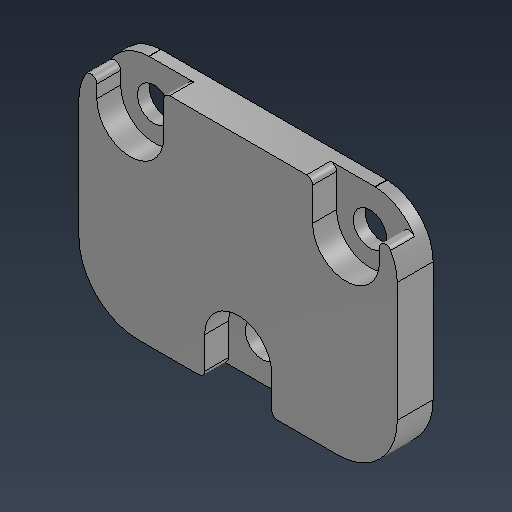
# Autodesk Inventor part: LunasCover
Saved by Autodesk Inventor 2026.2 (Build 302298010, 298A)
## iProperties
Created: 2026-04-20
Part Number: LunasCover
Material: Nylon 6/6
Document SubType Name: Modeling
Designer: szymo
Density: 1.13 g/cm^3
Appearance: Nylon 6(1)
Author: szymo
Autodesk Inventor part; units mm, degrees
ref_plane "YZ Plane" through (0, 0, 0) normal (1, 0, 0) x (0, 1, 0)
ref_plane "XZ Plane" through (0, 0, 0) normal (0, 1, 0) x (-1, 0, 0)
ref_plane "XY Plane" through (0, 0, 0) normal (0, 0, 1) x (1, 0, 0)
sketch "Sketch1" plane through (0, 0, 0) normal (0, 0, 1) x (1, 0, 0)
  circle A0 centre (0.0056, -6.3497) radius 1 projected
  circle A1 centre (-9.0264, 6.2307) radius 1 projected
  circle A2 centre (9.0376, 6.2307) radius 1 projected
  line L0 (9.4418, 9.5) -> (-9.4418, 9.5) projected
  arc A3 (-9.4806, 9.497) -> (-9.4418, 9.5) centre (-9.5, 9.9966) ccw projected
  arc A4 (-9.4806, 9.497) -> (-13.325, 5.5) centre (-9.325, 5.5) ccw projected
  line L1 (-13.325, -4.5) -> (-13.325, 5.5) projected
  arc A5 (-13.325, -4.5) -> (-8.325, -9.5) centre (-8.325, -4.5) ccw projected
  line L2 (8.325, -9.5) -> (-8.325, -9.5) projected
  arc A6 (8.325, -9.5) -> (13.325, -4.5) centre (8.325, -4.5) ccw projected
  line L3 (13.325, 5.5) -> (13.325, -4.5) projected
  arc A7 (13.325, 5.5) -> (9.4806, 9.497) centre (9.325, 5.5) ccw projected
  arc A8 (9.4418, 9.5) -> (9.4806, 9.497) centre (9.5, 9.9966) ccw projected
  point P0 (0, 0)
extrude "Extrusion1" add sketch "Sketch1" along normal blind 3
sketch "Sketch2" plane through (0, 0, 3) normal (0, 0, -1) x (-1, 0, 0)
  circle A0 centre (9.0264, 6.2307) radius 1 projected
  circle A1 centre (-0.0056, -6.3497) radius 1 projected
  circle A2 centre (-9.0376, 6.2307) radius 1 projected
  point P0 (0, 0)
hole "Hole1" at (-9.0264, 6.2307, 3) at (0.0056, -6.3497, 3) at (9.0376, 6.2307, 3) direction (0, 0, -1) diameter 2.8 depth 12 counterbore diameter 5.6 counterbore depth 2
sketch "Sketch3" plane through (0, 0, 3) normal (0, 0, 1) x (1, 0, 0)
  circle A0 centre (9.0376, 6.2307) radius 2.8 projected
  circle A1 centre (0.0056, -6.3497) radius 2.8 projected
  circle A2 centre (-9.0264, 6.2307) radius 2.8 projected
  arc A3 (9.4418, 9.5) -> (9.4806, 9.497) centre (9.5, 9.9966) ccw projected
  line L0 (9.4418, 9.5) -> (-9.4418, 9.5) projected
  arc A4 (-9.4806, 9.497) -> (-9.4418, 9.5) centre (-9.5, 9.9966) ccw projected
  arc A5 (-9.4806, 9.497) -> (-13.325, 5.5) centre (-9.325, 5.5) ccw projected
  line L1 (-13.325, 5.5) -> (-13.325, -4.5) projected
  arc A6 (-13.325, -4.5) -> (-8.325, -9.5) centre (-8.325, -4.5) ccw projected
  line L2 (-8.325, -9.5) -> (8.325, -9.5) projected
  arc A7 (8.325, -9.5) -> (13.325, -4.5) centre (8.325, -4.5) ccw projected
  line L3 (13.325, -4.5) -> (13.325, 5.5) projected
  arc A8 (13.325, 5.5) -> (9.4806, 9.497) centre (9.325, 5.5) ccw projected
  line L4 (-6.2264, 6.2307) -> (-6.2264, 9.5)
  line L5 (-11.8264, 6.2307) -> (-11.8264, 8.6214)
  circle A9 centre (-9.0264, 6.2307) radius 2.8 projected
  line L6 (6.2376, 6.2307) -> (6.2376, 9.5)
  line L7 (11.8376, 6.2307) -> (11.8376, 8.6123)
  line L8 (2.8056, -6.3497) -> (2.8056, -9.5)
  line L9 (-2.7944, -6.3497) -> (-2.7944, -9.5)
  point P0 (0, 0)
  constraints: 12 end point, 8 point on circle, 7 tangent, 4 perpendicular, 4 point on line, 1 parallel, 1 vertical
extrude "Extrusion2" cut sketch "Sketch3" against normal up to surface (2 mm away) contours A0 L6 L0 A3 A8 L7 | L4 A2 L5 A5 A4 L0 | L2 L9 A1 L8
fillet "Fillet1" radius 0.5 6 edges at (-11.8264, 8.6214, 2) (-6.2264, 9.5, 2) (6.2376, 9.5, 2) (11.8376, 8.6123, 2) (-2.7944, -9.5, 2) (2.8056, -9.5, 2)
body "Solid1"
